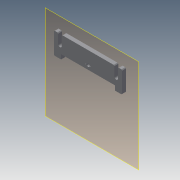
# Autodesk Inventor part: Lower Bracket
Saved by Autodesk Inventor 2014 SP1 (Build 180222100, 222)
## iProperties
Created: 2014-04-09
Part Number: Lower Bracket
Material: Generic
Document SubType Name: Modeling
Designer: tom
Density: 1 g/cm^3
Appearance: Default
Author: tom
Autodesk Inventor part; units mm, degrees
ref_plane "YZ Plane" through (0, 0, 0) normal (1, 0, 0) x (0, 1, 0)
ref_plane "XZ Plane" through (0, 0, 0) normal (0, 1, 0) x (-1, 0, 0)
ref_plane "XY Plane" through (0, 0, 0) normal (0, 0, 1) x (1, 0, 0)
ref_plane "Work Plane1" through (82.6105, 192.6947, -14.7678) normal (0, 0, 1) x (1, 0, 0)
sketch "Sketch1" plane through (82.6105, 192.6947, -14.7678) normal (0, 0, 1) x (1, 0, 0)
  line L0 (76.2, 79.375) -> (76.2, 31.115)
  arc A0 (-66.9925, 57.785) -> (-58.7375, 57.785) centre (-62.865, 57.785) ccw
  line L1 (-66.9925, 57.785) -> (-66.9925, 79.375)
  line L2 (-58.7375, 57.785) -> (-58.7375, 79.375)
  line L3 (-76.2, 79.375) -> (-66.9925, 79.375)
  line L4 (0, 79.375) -> (0, 48.4751) construction
  line L5 (58.7375, 57.785) -> (58.7375, 79.375)
  line L6 (66.9925, 57.785) -> (66.9925, 79.375)
  arc A1 (58.7375, 57.785) -> (66.9925, 57.785) centre (62.865, 57.785) ccw
  line L7 (-58.7375, 79.375) -> (58.7375, 79.375)
  line L8 (66.9925, 79.375) -> (76.2, 79.375)
  line L9 (-60.325, 41.275) -> (-60.325, 31.115)
  line L10 (-60.325, 41.275) -> (60.325, 41.275)
  line L11 (60.325, 41.275) -> (60.325, 31.115)
  line L12 (-76.2, 79.375) -> (-76.2, 31.115)
  circle A2 centre (0, 50.275) radius 3.5
  circle A3 centre (5.5, 50.275) radius 1
  circle A4 centre (-5.5, 50.275) radius 1
  line L13 (-60.325, 31.115) -> (-76.2, 31.115)
  line L14 (60.325, 31.115) -> (76.2, 31.115)
  point P0 (-82.6105, -192.6947)
  point P1 (0, 0)
  dimension "d1" = 76.2
  dimension "d4" = 8.255
  dimension "d10" = 152.4
  dimension "d11" = 7
  dimension "d12" = 9
  dimension "d13" = 2
  dimension "d14" = 5.5
  dimension "d15" = 2
  dimension "d16" = 5.5
  dimension "d17" = 57.785
  constraints: 30 end point, 11 perpendicular, 5 centre point, 5 symmetric about line, 4 point on circle, 3 horizontal, 2 tangent, 1 midpoint, 1 point on line, 2 other
  measures "d1" distance from line of point (0, 0) L0
  measures "d4" diameter of A0
  measures "d10" distance between parallel lines of L0 L12
  measures "d11" diameter of A2
  measures "d12" distance from line of L10 A2.centre
  measures "d13" diameter of A3
  measures "d14" distance of A3.centre A2.centre
  measures "d15" diameter of A4
  measures "d16" distance of A4.centre A2.centre
  measures "d17" vertical distance of point (0, 0) A0.centre
extrude "Extrusion1" add sketch "Sketch1" along normal blind 8.66
chamfer "Chamfer1" distance 1.5875 angle 45 8 edges at (158.8105, 223.8097, -10.4378) (141.348, 272.0697, -10.4378) (158.8105, 272.0697, -10.4378) (6.4105, 223.8097, -10.4378) (6.4105, 272.0697, -10.4378) (15.618, 272.0697, -10.4378) (23.873, 272.0697, -10.4378) (149.603, 272.0697, -10.4378)
equation "\"d1\" = 0.5 * d10"
body "Solid1"
